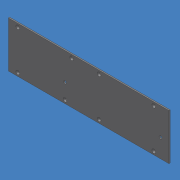
# Autodesk Inventor part: cRIO-FRC BackPlate
Saved by Autodesk Inventor 2011 (Build 150239000, 239)
## iProperties
Category: FRC Parts
Manager: Ed Sparks
Company: FirstCadLibrary
Shininess: 64.0
Length Units: 11272
Angle Units: 11279
Time Units: 11290
Mass Units: 11286
Length Display Precision: 3
Angle Display Precision: 2
Compacted: True
Part Number: cRIO-FRC BackPlate
Document SubType Name: Modeling
Created: 2008-12-10
Designer: Ed Sparks
Project: FIRST
Catalog Web Link: www.firstcadlibrary.com
Engineer: Ed Sparks
Material: Aluminum-Casting
Density: 2.61 g/cm^3
Density: 0.0
Volumn: 0.0
Area: 0.0
PropertySet Name: Model Information
Control State: 0
Master: False
Checked Out: False
Author: Ed Sparks
Keywords: FIRST
Autodesk Inventor part; units mm, degrees
ref_plane "YZ Plane" through (0, 0, 0) normal (1, 0, 0) x (0, 1, 0)
ref_plane "XZ Plane" through (0, 0, 0) normal (0, 1, 0) x (-1, 0, 0)
ref_plane "XY Plane" through (0, 0, 0) normal (0, 0, 1) x (1, 0, 0)
sketch "Sketch1" plane through (0, 0, 0) normal (0, 0, 1) x (1, 0, 0)
  line L0 (-138.811, 39.7129) -> (138.811, 39.7129)
  line L1 (138.811, 39.7129) -> (138.811, -39.7129)
  line L2 (138.811, -39.7129) -> (-138.811, -39.7129)
  line L3 (-138.811, -39.7129) -> (-138.811, 39.7129)
  line L4 (0, 0) -> (0, 39.7129) construction
  line L5 (0, 0) -> (0, -39.7129) construction
  line L6 (0, 0) -> (-138.811, 0) construction
  line L7 (0, 0) -> (138.811, 0) construction
  dimension "d0" = 277.622
  dimension "d1" = 79.4258
  constraints: 16 end point, 4 midpoint, 2 collinear, 2 parallel, 1 horizontal, 1 perpendicular, 1 other
  measures "d0" distance of L0.start L0.end
  measures "d1" distance of L2.end L0.start
extrude "Extrusion1" add sketch "Sketch1" along normal mid plane 2.2098
sketch "Sketch2" plane through (0, 0, 1.1049) normal (0, 0, 1) x (1, 0, 0)
  line L0 (138.811, 39.7129) -> (138.811, -39.7129) projected
  line L1 (-138.811, 39.7129) -> (138.811, 39.7129) projected
  line L2 (-138.811, -39.7129) -> (-138.811, 39.7129) projected
  line L3 (138.811, -39.7129) -> (-138.811, -39.7129) projected
  circle A0 centre (-122.5042, 33.9217) radius 3.3401
  circle A1 centre (-29.4894, 33.9217) radius 3.3401
  circle A2 centre (18.0848, 33.9217) radius 3.3401
  circle A3 centre (112.5728, 33.9217) radius 3.3401
  circle A4 centre (-122.5042, -33.9217) radius 3.3401
  circle A5 centre (-40.9702, -33.9217) radius 3.3401
  circle A6 centre (18.0848, -33.9217) radius 3.3401
  circle A7 centre (112.5728, -33.9217) radius 3.3401
  dimension "d4" = 16.3068
  dimension "d5" = 5.7912
  dimension "d6" = 5.7912
  dimension "d7" = 26.2382
  dimension "d8" = 120.7262
  dimension "d9" = 168.3004
  dimension "d10" = 179.7812
  dimension "d11" = 6.6802
  constraints: 8 centre point, 8 coincident, 7 equal radius, 6 horizontal alignment, 3 vertical alignment
  measures "d4" distance from line of L2 point (-122.504, 33.922)
  measures "d5" distance from line of L1 point (-122.504, 33.922)
  measures "d6" distance from line of point (-122.504, -33.922) L3
  measures "d7" distance from line of point (112.573, 33.922) L0
  measures "d8" distance from line of L0 point (18.085, 33.922)
  measures "d9" distance from line of point (-29.489, 33.922) L0
  measures "d10" distance from line of L0 point (-40.97, -33.922)
  measures "d11" diameter of A0
extrude "Extrusion2" add sketch "Sketch2" against normal blind 4.5974 contours A0 | A1 | A2 | A3 | A4 | A5 | A6 | A7
sketch "Sketch3" plane through (0, 0, 1.1049) normal (0, 0, 1) x (1, 0, 0)
  circle A0 centre (-122.5042, 33.9217) radius 3.3401 projected
  circle A1 centre (-122.5042, -33.9217) radius 3.3401 projected
  circle A2 centre (-29.4894, 33.9217) radius 3.3401 projected
  circle A3 centre (-40.9702, -33.9217) radius 3.3401 projected
  circle A4 centre (18.0848, -33.9217) radius 3.3401 projected
  circle A5 centre (18.0848, 33.9217) radius 3.3401 projected
  circle A6 centre (112.5728, 33.9217) radius 3.3401 projected
  circle A7 centre (112.5728, -33.9217) radius 3.3401 projected
hole "Hole1" at (-122.5042, 33.9217, 1.1049) at (-29.4894, 33.9217, 1.1049) at (18.0848, 33.9217, 1.1049) at (112.5728, 33.9217, 1.1049) at (112.5728, -33.9217, 1.1049) at (18.0848, -33.9217, 1.1049) at (-40.9702, -33.9217, 1.1049) at (-122.5042, -33.9217, 1.1049) direction (0, 0, -1) diameter 3.1496 end through all countersink diameter 6.731 countersink angle 82
sketch "Sketch4" plane through (0, 0, 1.1049) normal (0, 0, 1) x (1, 0, 0)
  line L0 (138.811, 39.7129) -> (138.811, -39.7129) projected
  line L1 (-138.811, 39.7129) -> (138.811, 39.7129) projected
  point P0 (-40.9702, -7.6581)
  point P1 (124.1298, -7.6581)
  dimension "d21" = 47.371
  dimension "d22" = 14.6812
  dimension "d23" = 165.1
  constraints: 1 horizontal alignment
  measures "d21" distance from line of L1 point (-40.97, -7.658)
  measures "d22" distance from line of L0 point (124.13, -7.658)
  measures "d23" distance of point (-40.97, -7.658) point (124.13, -7.658)
hole "Hole2" at (-40.9702, -7.6581, 1.1049) at (124.1298, -7.6581, 1.1049) direction (0, 0, -1) diameter 5.2324 end through all
body "Solid1"
